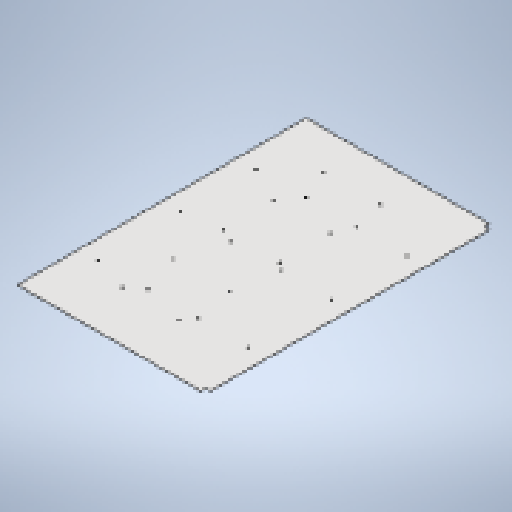
# Autodesk Inventor part: GnG L.1 floor sheet
Saved by Autodesk Inventor 2025.3 (Build 293356030, 356C)
## iProperties
Created: 2025-10-28
Part Number: GnG L.1 floor sheet
Material: Stainless Steel
Document SubType Name: Sheet Metal
Designer: admin
Mass: 280.619 g
Surface Area: 364.406 cm^2
Volume: 35.0774 cm^3
Density: 8 g/cm^3
Sheet Metal Rule: AISI304 3mm Die 32
Sheet Metal Width: 1500,000 mm
Sheet Metal Length: 2300,000 mm
Sheet Metal Area: 3450000,000 mm^2
Appearance: Default
Stock Number: L 1
Flat Pattern Width: 150 cm
Flat Pattern Length: 230 cm
Flat Pattern Area: 34500 cm^2
Author: admin
Autodesk Inventor part; units mm, degrees
ref_plane "YZ Plane" through (0, 0, 0) normal (1, 0, 0) x (0, 1, 0)
ref_plane "XZ Plane" through (0, 0, 0) normal (0, 1, 0) x (-1, 0, 0)
ref_plane "XY Plane" through (0, 0, 0) normal (0, 0, 1) x (1, 0, 0)
sketch "Sketch1" plane through (0, 0, 0) normal (0, 0, 1) x (1, 0, 0)
  line L0 (0, 0) -> (-1500, 0)
  line L1 (-1500, 0) -> (-1500, -2300)
  line L2 (-1500, -2300) -> (0, -2300)
  line L3 (0, -2300) -> (0, 0)
  line L4 (0, 0) -> (-40, 0)
  line L5 (-40, 0) -> (-40, -40)
  line L6 (-40, -40) -> (0, -40)
  line L7 (0, -40) -> (0, 0)
  line L8 (0, -2300) -> (-40, -2300)
  line L9 (-40, -2300) -> (-40, -2260)
  line L10 (-40, -2260) -> (0, -2260)
  line L11 (0, -2260) -> (0, -2300)
  point P0 (0, -40)
  point P1 (-40, -2300)
  point P2 (0, -2260)
  dimension "d22" = 1500
  dimension "d23" = 2300
  dimension "d24" = 40
  dimension "d25" = 40
  measures "d22" distance of L2.end L1.end
  measures "d23" distance of L1.end L0.end
  measures "d24" distance of L6.end L5.end
  measures "d25" distance of L5.end L4.end
extrude "Plate1" add sketch "Sketch1" along normal blind 3 contours L5 L6 L3 L10 L9 L2 L1 L0
sketch "Sketch5" plane through (0, 0, 3) normal (0, 0, 1) x (1, 0, 0)
  line L0 (-1500, -2300) -> (-1500, 0) projected
  line L1 (-40, -2300) -> (-1500, -2300) projected
  line L2 (-40, -2260) -> (-40, -2300) projected
  line L3 (0, -2260) -> (-40, -2260) projected
  line L4 (0, -40) -> (0, -2260) projected
  line L5 (-40, -40) -> (0, -40) projected
  line L6 (-40, 0) -> (-40, -40) projected
  line L7 (-1500, 0) -> (-40, 0) projected
  line L8 (-1400, 0) -> (-1396, 0)
  line L9 (-1396, 0) -> (-1396, -2)
  line L10 (-1396, -2) -> (-1400, -2)
  line L11 (-1400, -2) -> (-1400, 0)
  line L12 (-1384, 0) -> (-1380, 0)
  line L13 (-1380, 0) -> (-1380, -2)
  line L14 (-1380, -2) -> (-1384, -2)
  line L15 (-1384, -2) -> (-1384, 0)
  line L16 (-1392, 0) -> (-1388, 0)
  line L17 (-1388, 0) -> (-1388, -2)
  line L18 (-1388, -2) -> (-1392, -2)
  line L19 (-1392, -2) -> (-1392, 0)
  line L20 (-1500, 0) -> (-40, 0) projected
  line L21 (-1396, -1) -> (-1392, -1)
  line L22 (-1376, 0) -> (-1373, 0)
  line L23 (-1388, -1) -> (-1384, -1)
  line L24 (-1376, 0) -> (-1375.4231, -1.3846)
  arc A0 (-1375.4231, -1.3846) -> (-1373.5769, -1.3846) centre (-1374.5, -1) ccw
  line L25 (-1373.5769, -1.3846) -> (-1373, 0)
  line L26 (-1380, 0) -> (-1376, 0)
  line L27 (-1369, 0) -> (-1365, 0)
  line L28 (-1365, 0) -> (-1365, -5)
  line L29 (-1365, -5) -> (-1369, -5)
  line L30 (-1369, -5) -> (-1369, 0)
  line L31 (-1353, 0) -> (-1349, 0)
  line L32 (-1349, 0) -> (-1349, -5)
  line L33 (-1349, -5) -> (-1353, -5)
  line L34 (-1353, -5) -> (-1353, 0)
  line L35 (-1361, 0) -> (-1357, 0)
  line L36 (-1357, 0) -> (-1357, -5)
  line L37 (-1357, -5) -> (-1361, -5)
  line L38 (-1361, -5) -> (-1361, 0)
  line L39 (-1365, -2.5) -> (-1361, -2.5)
  line L40 (-1357, -2.5) -> (-1353, -2.5)
  line L41 (-1373, 0) -> (-1369, 0)
  line L42 (-40, 0) -> (-1500, 0) projected
  circle A1 centre (-1405, 0) radius 2.5
  point P0 (0, 0)
  point P1 (-1382, 0)
  point P2 (-1390, 0)
  point P3 (-1374.5, 0)
  point P4 (-1396, 0)
  point P5 (-1351, 0)
  point P6 (-1359, 0)
  point P7 (-1367, 0)
  point P8 (-1407.5, 0)
  point P9 (-1402.5, 0)
  point P10 (-1407.5, 0)
  point P11 (-1402.5, 0)
  dimension "d34" = 4
  dimension "d35" = 2
  dimension "d36" = 1
  dimension "d37" = 100
  dimension "d40" = 3
  dimension "d41" = 4
  dimension "d42" = 5
  dimension "d43" = 5
  dimension "d44" = 5
  constraints: 66 end point, 14 midpoint, 12 parallel, 10 equal length, 10 horizontal, 6 perpendicular, 4 collinear, 3 tangent, 2 centre point, 2 point on circle, 1 point on line, 1 vertical alignment, 8 other
  measures "d34" distance of L9.end L10.end
  measures "d35" distance of L10.end L8.start
  measures "d36" radius of A0
  measures "d37" distance between parallel lines of L0 L11
  measures "d40" distance of L22.start L22.end
  measures "d41" distance of L29.start L29.end
  measures "d42" distance of L29.end L27.start
  measures "d43" diameter of A1
  measures "d44" distance of A1.centre L8.start
extrude "Cut1" cut sketch "Sketch5" against normal blind 3 contours L7 A1 | L7 L9 L10 L11 picked at (-1405.7379, -0.3873)
sketch "Sketch6" plane through (0, 0, 0) normal (0, 0, -1) x (-1, 0, 0)
  line L0 (1400, 0) -> (1400, -2) construction
  line L1 (1400, -2) -> (1396, -2) construction
  line L2 (1396, -2) -> (1396, 0) construction
  line L3 (40, 0) -> (1396, 0) construction
  line L4 (40, -40) -> (40, 0) construction
  line L5 (0, -40) -> (40, -40) construction
  line L6 (0, -2260) -> (0, -40) construction
  line L7 (40, -2260) -> (0, -2260) construction
  line L8 (40, -2300) -> (40, -2260) construction
  line L9 (1500, -2300) -> (40, -2300) construction
  line L10 (1500, 0) -> (1500, -2300) construction
  line L11 (1407.5, 0) -> (1500, 0) construction
  arc A0 (1402.5, 0) -> (1407.5, 0) centre (1405, 0) ccw construction
  line L12 (1400, 0) -> (1402.5, 0) construction
  line L13 (1060, 0) -> (1060, -2300) construction
  line L14 (610, 0) -> (610, -2300) construction
  line L15 (1500, -1810) -> (0, -1810) construction
  line L16 (1500, -1150) -> (0, -1150) construction
  line L17 (1500, -550) -> (0, -550) construction
  circle A1 centre (1350, -550) radius 7.5
  circle A2 centre (1350, -1150) radius 7.5
  circle A3 centre (1350, -1810) radius 7.5
  circle A4 centre (1060, -1900) radius 7.5
  circle A5 centre (610, -1900) radius 7.5
  circle A6 centre (610, -1500) radius 7.5
  circle A7 centre (1060, -1500) radius 7.5
  circle A8 centre (610, -1100) radius 7.5
  circle A9 centre (1060, -1100) radius 7.5
  circle A10 centre (610, -700) radius 7.5
  circle A11 centre (1060, -700) radius 7.5
  circle A12 centre (610, -300) radius 7.5
  circle A13 centre (1060, -300) radius 7.5
  circle A14 centre (610, 100) radius 7.5
  circle A15 centre (1060, 100) radius 7.5
  circle A16 centre (610, 500) radius 7.5
  circle A17 centre (1060, 500) radius 7.5
  circle A18 centre (610, 900) radius 7.5
  circle A19 centre (1060, 900) radius 7.5
  circle A20 centre (610, 1300) radius 7.5
  circle A21 centre (1060, 1300) radius 7.5
  circle A22 centre (610, 1700) radius 7.5
  circle A23 centre (1060, 1700) radius 7.5
  circle A24 centre (610, 2100) radius 7.5
  circle A25 centre (1060, 2100) radius 7.5
  circle A26 centre (950, -1810) radius 7.5
  circle A27 centre (950, -1150) radius 7.5
  circle A28 centre (950, -550) radius 7.5
  circle A29 centre (550, -1810) radius 7.5
  circle A30 centre (550, -1150) radius 7.5
  circle A31 centre (550, -550) radius 7.5
  circle A32 centre (150, -1810) radius 7.5
  circle A33 centre (150, -1150) radius 7.5
  circle A34 centre (150, -550) radius 7.5
  circle A35 centre (-250, -1810) radius 7.5
  circle A36 centre (-250, -1150) radius 7.5
  circle A37 centre (-250, -550) radius 7.5
  circle A38 centre (-650, -1810) radius 7.5
  circle A39 centre (-650, -1150) radius 7.5
  circle A40 centre (-650, -550) radius 7.5
  circle A41 centre (-1050, -1810) radius 7.5
  circle A42 centre (-1050, -1150) radius 7.5
  circle A43 centre (-1050, -550) radius 7.5
  point P0 (0, 0)
  dimension "d45" = 440
  dimension "d46" = 890
  dimension "d47" = 550
  dimension "d48" = 1150
  dimension "d49" = 1810
  dimension "d50" = 15
  dimension "d51" = 400
  dimension "d52" = 150
  dimension "d55" = 400
  dimension "d62" = 400
  constraints: 43 centre point, 13 point on line, 10 end point, 5 perpendicular, 4 equal radius, 2 midpoint, 2 vertical alignment, 1 horizontal, 1 horizontal alignment, 1 vertical, 76 other
  measures "d45" distance between parallel lines of L13 L10
  measures "d46" distance between parallel lines of L14 L10
  measures "d47" distance between parallel lines of L17 L3
  measures "d48" distance between parallel lines of L16 L3
  measures "d49" distance between parallel lines of L15 L3
  measures "d50" diameter of A4
  measures "d51" distance from line of A4.centre L9
  measures "d52" distance from line of A3.centre L10
  measures "d55" distance of A5.centre A6.centre
  measures "d62" distance of A3.centre A26.centre
extrude "Cut2" cut sketch "Sketch6" against normal blind 3
equation "\"d25\" = d24"
equation "\"d36\" = 0.25 * d34"
equation "\"d41\" = d34"
equation "\"d38\" = Thickness"
equation "\"d67\" = Thickness"
equation "\"d2\" = Thickness"
equation "\"BendReliefWidth\" = Thickness"
equation "\"BendReliefDepth\" = 0.5 * Thickness"
equation "\"CornerReliefSize\" = 4 * Thickness"
equation "\"MinimumRemnant\" = 2 * Thickness"
equation "\"TransitionRadius\" = BendRadius"
equation "\"JacobiRadiusSize\" = BendRadius"
equation "\"GapSize\" = Thickness"
equation "\"Thickness\" = 3"
equation "\"BendRadius\" = 5"
body "Solid1"
